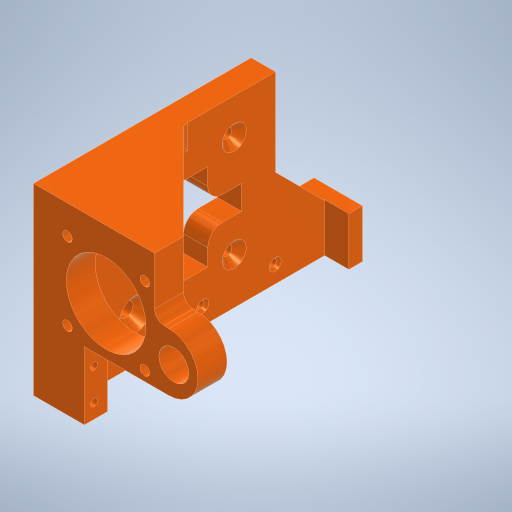
# Autodesk Inventor part: Z_motor_holder
Saved by Autodesk Inventor 2024.1 (Build 281209000, 209)
## iProperties
Created: 2023-09-27
Part Number: Z_motor_holder
Material: ABS Plastic
Document SubType Name: Modeling
Designer: l1534
Density: 1.06 g/cm^3
Appearance: Smooth - Light Orange
Author: l1534
Autodesk Inventor part; units mm, degrees
ref_plane "YZ Plane" through (0, 0, 0) normal (1, 0, 0) x (0, 1, 0)
ref_plane "XZ Plane" through (0, 0, 0) normal (0, 1, 0) x (-1, 0, 0)
ref_plane "XY Plane" through (0, 0, 0) normal (0, 0, 1) x (1, 0, 0)
sketch "Sketch1" plane through (0, 0, 0) normal (1, 0, 0) x (0, 1, 0)
  line L0 (-23.3447, 18.3788) -> (14.6553, 18.3788)
  line L1 (14.6553, 18.3788) -> (14.6553, -36.6212)
  line L2 (14.6553, -36.6212) -> (-23.3447, -36.6212)
  line L3 (-23.3447, -36.6212) -> (-23.3447, 18.3788)
  point P0 (0, 0)
  dimension "d0" = 38
  dimension "d1" = 55
  constraints: 8 end point, 2 parallel, 1 horizontal, 1 perpendicular
  measures "d0" distance of L0.start L0.end
  measures "d1" distance of L2.end L0.start
extrude "Extrusion1" add sketch "Sketch1" along normal blind 5
sketch "Sketch2" plane through (5, 0, 0) normal (1, 0, 0) x (0, 0, -1)
  line L0 (36.6212, 14.6553) -> (-18.3788, 14.6553) projected
  line L1 (-18.3788, 14.6553) -> (-12.3788, 14.6553)
  line L2 (-12.3788, 14.6553) -> (-12.3788, -9.3447)
  line L3 (-12.3788, -9.3447) -> (-18.3788, -9.3447)
  line L4 (-18.3788, -9.3447) -> (-18.3788, 14.6553)
  point P0 (0, 0)
  dimension "d4" = 24
  dimension "d5" = 6
  constraints: 8 end point, 2 parallel, 1 horizontal, 1 perpendicular
  measures "d4" distance of L3.end L0.end
  measures "d5" distance of L2.end L3.end
extrude "Extrusion2" add sketch "Sketch2" along normal blind 20
sketch "Sketch3" plane through (5, -9.3447, 12.3788) normal (0, 0, -1) x (-1, 0, 0)
  circle A0 centre (-10, 10) radius 8.25
  line L0 (-20, 0) -> (-20, 24) projected
  line L1 (0, 0) -> (-20, 0) projected
  circle A1 centre (-18, 2) radius 1
  circle A2 centre (-18, 18) radius 1
  circle A3 centre (-2, 2) radius 1
  circle A4 centre (-2, 18) radius 1
  point P0 (5, 9.3447)
  dimension "d8" = 16.5
  dimension "d9" = 10
  dimension "d10" = 10
  dimension "d11" = 2
  dimension "d12" = 2
  dimension "d13" = 2
  dimension "d14" = 2
  dimension "d15" = 8
  dimension "d16" = 8
  dimension "d17" = 8
  dimension "d18" = 8
  dimension "d19" = 8
  dimension "d20" = 8
  dimension "d21" = 8
  dimension "d22" = 8
  constraints: 5 centre point
  measures "d8" diameter of A0
  measures "d9" distance from line of L0 A0.centre
  measures "d10" distance from line of L1 A0.centre
  measures "d11" diameter of A1
  measures "d12" diameter of A2
  measures "d13" diameter of A3
  measures "d14" diameter of A4
  measures "d15" horizontal distance of A0.centre A1.centre
  measures "d16" horizontal distance of A0.centre A1.centre
  measures "d17" horizontal distance of A0.centre A2.centre
  measures "d18" horizontal distance of A0.centre A2.centre
  measures "d19" horizontal distance of A0.centre A3.centre
  measures "d20" horizontal distance of A0.centre A3.centre
  measures "d21" horizontal distance of A0.centre A4.centre
  measures "d22" horizontal distance of A0.centre A4.centre
extrude "Extrusion3" cut sketch "Sketch3" against normal through all
sketch "Sketch4" plane through (5, -9.3447, 12.3788) normal (0, 0, -1) x (-1, 0, 0)
  line L0 (-20, 24) -> (-20, 0) projected
  line L1 (0, 24) -> (0, 0) projected
  line L2 (-20, 24) -> (0, 24)
  line L3 (0, 24) -> (0, 21)
  line L4 (0, 21) -> (-20, 21)
  line L5 (-20, 21) -> (-20, 24)
  point P0 (5, 9.3447)
  dimension "d25" = 3
  constraints: 8 end point, 2 parallel, 1 horizontal, 1 perpendicular, 1 point on line
  measures "d25" distance between parallel lines of L2 L4
extrude "Extrusion4" add sketch "Sketch4" along normal blind 20
sketch "Sketch5" plane through (5, 11.6553, 12.3788) normal (0, -1, 0) x (1, 0, 0)
  line L0 (0, -20) -> (0, 0) projected
  line L1 (20, 6) -> (20, 0) projected
  line L2 (0, -20) -> (20, 0)
  line L3 (20, 0) -> (20, -20)
  line L4 (20, -20) -> (0, -20) projected
  line L5 (20, -20) -> (0, -20)
  point P0 (-5, -12.3788)
  constraints: 6 end point, 2 collinear
extrude "Extrusion5" cut sketch "Sketch5" against normal through all
fillet "Fillet1" radius 2 2 edges at (5, 11.6553, 2.3788) (5, 13.1553, -7.6212)
sketch "Sketch6" plane through (5, 0, 0) normal (1, 0, 0) x (0, 0, -1)
  circle A0 centre (1.6212, -3.3447) radius 1
  line L0 (36.6212, 14.6553) -> (8.4496, 14.6553) projected
  line L1 (36.6212, -23.3447) -> (36.6212, 14.6553) projected
  point P0 (0, 0)
  dimension "d31" = 2
  dimension "d32" = 18
  dimension "d33" = 35
  constraints: 1 centre point
  measures "d31" diameter of A0
  measures "d32" distance from line of L0 A0.centre
  measures "d33" distance from line of L1 A0.centre
extrude "Extrusion6" cut sketch "Sketch6" against normal through all
sketch "Sketch7" plane through (5, 0, 0) normal (1, 0, 0) x (0, 0, -1)
  circle A0 centre (-2.3788, -14.3447) radius 1.5
  circle A1 centre (-2.3788, 7.6553) radius 1.5
  circle A2 centre (1.6212, -3.3447) radius 1 projected
  point P0 (0, 0)
  dimension "d36" = 3
  dimension "d37" = 3
  dimension "d38" = 4
  dimension "d39" = 11
  dimension "d40" = 11
  dimension "d41" = 4
  constraints: 2 centre point
  measures "d36" diameter of A0
  measures "d37" diameter of A1
  measures "d38" horizontal distance of A2.centre A0.centre
  measures "d39" vertical distance of A2.centre A0.centre
  measures "d40" vertical distance of A2.centre A1.centre
  measures "d41" horizontal distance of A2.centre A1.centre
extrude "Extrusion7" cut sketch "Sketch7" against normal through all contours A0 | A1
chamfer "Chamfer1" distance 1.5 angle 45 1 edges at (5, -3.3447, -0.6212)
chamfer "Chamfer2" distance 1.9 angle 45 2 edges at (5, -14.3447, 3.8788) (5, 7.6553, 3.8788)
sketch "Sketch8" plane through (5, 0, 0) normal (1, 0, 0) x (0, 0, -1)
  line L0 (36.6212, 14.6553) -> (-18.3788, 14.6553) projected
  line L1 (36.6212, 14.6553) -> (26.6212, 14.6553)
  line L2 (26.6212, 14.6553) -> (26.6212, -13.3447)
  line L3 (26.6212, -13.3447) -> (36.6212, -13.3447)
  line L4 (36.6212, -13.3447) -> (36.6212, 14.6553)
  point P0 (0, 0)
  dimension "d50" = 28
  dimension "d51" = 10
  constraints: 8 end point, 2 parallel, 1 horizontal, 1 perpendicular
  measures "d50" distance of L1.end L2.end
  measures "d51" distance between parallel lines of L4 L2
extrude "Extrusion8" cut sketch "Sketch8" against normal through all
chamfer "Chamfer3" distance 10 angle 45 1 edges at (2.5, -13.3447, -26.6212)
sketch "Sketch9" plane through (5, 0, 0) normal (1, 0, 0) x (0, 0, -1)
  circle A0 centre (18.1212, -13.8447) radius 1
  circle A1 centre (18.1212, 7.1553) radius 1
  line L0 (26.6212, 14.6553) -> (8.4496, 14.6553) projected
  line L1 (36.6212, -23.3447) -> (36.6212, -13.3447) projected
  line L2 (-18.3788, -23.3447) -> (36.6212, -23.3447) projected
  point P0 (0, 0)
  dimension "d57" = 2
  dimension "d58" = 2
  dimension "d59" = 7.5
  dimension "d60" = 18.5
  dimension "d61" = 9.5
  dimension "d62" = 18.5
  constraints: 2 centre point
  measures "d57" diameter of A0
  measures "d58" diameter of A1
  measures "d59" distance from line of L0 A1.centre
  measures "d60" distance from line of L1 A1.centre
  measures "d61" distance from line of L2 A0.centre
  measures "d62" distance from line of L1 A0.centre
extrude "Extrusion9" cut sketch "Sketch9" against normal through all
chamfer "Chamfer4" distance 1.5 angle 45 2 edges at (5, -13.8447, -17.1212) (5, 7.1553, -17.1212)
sketch "Sketch10" plane through (5, 0, 0) normal (1, 0, 0) x (0, 0, -1)
  circle A0 centre (26.6212, -19.8447) radius 0.75
  circle A1 centre (11.6212, -19.8447) radius 0.75
  circle A2 centre (-3.3788, -19.8447) radius 0.75
  line L0 (-18.3788, -23.3447) -> (36.6212, -23.3447) projected
  line L1 (36.6212, -23.3447) -> (36.6212, -13.3447) projected
  line L2 (-18.3788, -9.3447) -> (-18.3788, -23.3447) projected
  point P0 (0, 0)
  dimension "d68" = 1.5
  dimension "d69" = 1.5
  dimension "d70" = 1.5
  dimension "d71" = 3.5
  dimension "d72" = 10
  dimension "d73" = 3.5
  dimension "d74" = 15
  dimension "d76" = 3.5
  dimension "d95" = 15
  constraints: 3 centre point
  measures "d68" diameter of A2
  measures "d69" diameter of A1
  measures "d70" diameter of A0
  measures "d71" distance from line of L0 A0.centre
  measures "d72" distance from line of L1 A0.centre
  measures "d73" distance from line of L0 A1.centre
  measures "d74" distance of A0.centre A1.centre
  measures "d76" distance from line of L0 A2.centre
  measures "d95" distance of A1.centre A2.centre
extrude "Extrusion10" cut sketch "Sketch10" against normal through all
sketch "Sketch15" plane through (5, 0, 0) normal (1, 0, 0) x (0, 0, -1)
  line L0 (36.6212, -23.3447) -> (36.6212, -13.3447) projected
  line L1 (36.6212, -23.3447) -> (39.6212, -23.3447)
  line L2 (39.6212, -23.3447) -> (39.6212, -13.3447)
  line L3 (39.6212, -13.3447) -> (36.6212, -13.3447)
  line L4 (36.6212, -13.3447) -> (36.6212, -23.3447)
  point P0 (0, 0)
  dimension "d96" = 3
  dimension "d97" = 10
  constraints: 8 end point, 2 parallel, 1 horizontal, 1 perpendicular
  measures "d96" distance of L2.end L3.end
  measures "d97" distance of L1.end L2.end
extrude "Extrusion15" add sketch "Sketch15" against normal up to surface (5 mm away)
sketch "Sketch16" plane through (5, 0, 0) normal (1, 0, 0) x (0, 0, -1)
  line L0 (-18.3788, -23.3447) -> (39.6212, -23.3447) projected
  line L1 (39.6212, -13.3447) -> (36.6212, -13.3447) projected
  line L2 (39.6212, -23.3447) -> (36.8212, -23.3447)
  line L3 (36.8212, -23.3447) -> (36.8212, -13.3447)
  line L4 (36.8212, -13.3447) -> (39.6212, -13.3447)
  line L5 (39.6212, -13.3447) -> (39.6212, -23.3447)
  point P0 (0, 0)
  dimension "d100" = 2.8
  constraints: 8 end point, 2 parallel, 1 horizontal, 1 perpendicular, 1 point on line
  measures "d100" distance between parallel lines of L5 L3
extrude "Extrusion16" add sketch "Sketch16" along normal blind 5
sketch "Sketch17" plane through (5, 0, 0) normal (1, 0, 0) x (0, 0, -1)
  line L0 (-18.3788, -23.3447) -> (39.6212, -23.3447) projected
  line L1 (-12.3788, -9.3447) -> (-18.3788, -9.3447) projected
  line L2 (-18.3788, -23.3447) -> (-13.5788, -23.3447)
  line L3 (-13.5788, -23.3447) -> (-13.5788, -9.3447)
  line L4 (-13.5788, -9.3447) -> (-18.3788, -9.3447)
  line L5 (-18.3788, -9.3447) -> (-18.3788, -23.3447)
  point P0 (0, 0)
  dimension "d103" = 4.8
  constraints: 8 end point, 2 parallel, 1 horizontal, 1 perpendicular, 1 point on line
  measures "d103" distance between parallel lines of L5 L3
extrude "Extrusion17" add sketch "Sketch17" along normal blind 5.5
sketch "Sketch18" plane through (10.5, 0, 0) normal (1, 0, 0) x (0, 0, -1)
  circle A0 centre (-16.3788, -20.3447) radius 0.75
  circle A1 centre (-16.3788, -13.8447) radius 0.75
  line L0 (-18.3788, -23.3447) -> (-13.5788, -23.3447) projected
  line L1 (-18.3788, -9.3447) -> (-18.3788, -23.3447) projected
  point P0 (0, 0)
  point P1 (-15.9788, -23.3447)
  dimension "d106" = 1.5
  dimension "d107" = 1.5
  dimension "d108" = 6.5
  dimension "d109" = 3
  dimension "d110" = 2
  dimension "d111" = 2
  constraints: 2 centre point, 1 midpoint
  measures "d106" diameter of A0
  measures "d107" diameter of A1
  measures "d108" distance of A1.centre A0.centre
  measures "d109" vertical distance of point (-15.979, -23.345) A0.centre
  measures "d110" distance from line of L1 A1.centre
  measures "d111" distance from line of L1 A0.centre
extrude "Extrusion18" cut sketch "Sketch18" against normal through all
sketch "Sketch19" plane through (5, 0, 0) normal (1, 0, 0) x (0, 0, -1)
  line L0 (7.6212, -13.3447) -> (12.6212, -13.3447)
  line L1 (12.6212, -13.3447) -> (12.6212, 4.6553)
  line L2 (12.6212, 4.6553) -> (7.6212, 4.6553)
  line L3 (7.6212, 4.6553) -> (7.6212, -13.3447)
  line L4 (26.6212, 14.6553) -> (8.4496, 14.6553) projected
  line L5 (-13.5788, -23.3447) -> (36.8212, -23.3447) projected
  line L6 (26.6212, -3.3447) -> (26.6212, 14.6553) projected
  point P0 (0, 0)
  dimension "d114" = 5
  dimension "d115" = 10
  dimension "d116" = 10
  dimension "d117" = 14
  constraints: 8 end point, 2 parallel, 1 horizontal, 1 perpendicular
  measures "d114" distance of L1.end L2.end
  measures "d115" distance between parallel lines of L4 L2
  measures "d116" distance between parallel lines of L5 L0
  measures "d117" distance between parallel lines of L6 L1
extrude "Extrusion19" cut sketch "Sketch19" against normal through all
chamfer "Chamfer5" distance 0.5 angle 45 3 edges at (5, -19.8447, 4.1288) (5, -19.8447, -10.8712) (5, -19.8447, -25.8712)
sketch "Sketch20" plane through (25, 0, 0) normal (1, 0, 0) x (0, 0, -1)
  line L0 (-12.3788, -9.3447) -> (-13.5788, -9.3447) projected
  line L1 (-18.3788, 14.6553) -> (-18.3788, -9.3447) projected
  line L2 (-12.3788, -9.3447) -> (-18.3788, -9.3447)
  line L3 (-18.3788, -9.3447) -> (-18.3788, 2.6553)
  line L4 (-18.3788, 2.6553) -> (-12.3788, 2.6553)
  line L5 (-12.3788, 2.6553) -> (-12.3788, -9.3447)
  point P0 (0, 0)
  dimension "d123" = 12
  constraints: 8 end point, 2 parallel, 1 horizontal, 1 midpoint, 1 perpendicular
  measures "d123" distance between parallel lines of L2 L4
extrude "Extrusion20" add sketch "Sketch20" along normal blind 9
sketch "Sketch21" plane through (0, -23.3447, 18.3788) normal (0, 0, 1) x (1, 0, 0)
  circle A0 centre (29, 20) radius 3.1
  line L0 (25, 26) -> (34, 26) projected
  line L1 (34, 26) -> (34, 14) projected
  point P0 (0, 23.3447)
  dimension "d126" = 6.2
  dimension "d127" = 6
  dimension "d128" = 5
  constraints: 1 centre point
  measures "d126" diameter of A0
  measures "d127" distance from line of L0 A0.centre
  measures "d128" distance from line of L1 A0.centre
extrude "Extrusion21" cut sketch "Sketch21" against normal through all
fillet "Fillet3" radius 6 2 edges at (34, -9.3447, 15.3788) (34, 2.6553, 15.3788)
sketch "Sketch22" plane through (5, 0, 0) normal (1, 0, 0) x (0, 0, -1)
  line L0 (12.6212, -13.3447) -> (12.6212, 4.6553) projected
  line L1 (12.6212, -6.8447) -> (19.6212, -6.8447)
  line L2 (19.6212, -6.8447) -> (19.6212, -1.8447)
  line L3 (19.6212, -1.8447) -> (12.6212, -1.8447)
  line L4 (12.6212, -1.8447) -> (12.6212, -6.8447)
  line L5 (7.6212, 4.6553) -> (12.6212, 4.6553) projected
  point P0 (0, 0)
  dimension "d134" = 5
  dimension "d135" = 6.5
  dimension "d136" = 7
  constraints: 8 end point, 2 parallel, 1 horizontal, 1 perpendicular, 1 point on line
  measures "d134" distance of L1.end L2.end
  measures "d135" distance between parallel lines of L5 L3
  measures "d136" distance of L1.start L1.end
extrude "Extrusion22" cut sketch "Sketch22" against normal through all
fillet "Fillet5" radius 3 2 edges at (2.5, -6.8447, -12.6212) (2.5, -1.8447, -12.6212)
fillet "Fillet6" radius 2 1 edges at (25, 2.6553, 15.3788)
body "Solid1"
